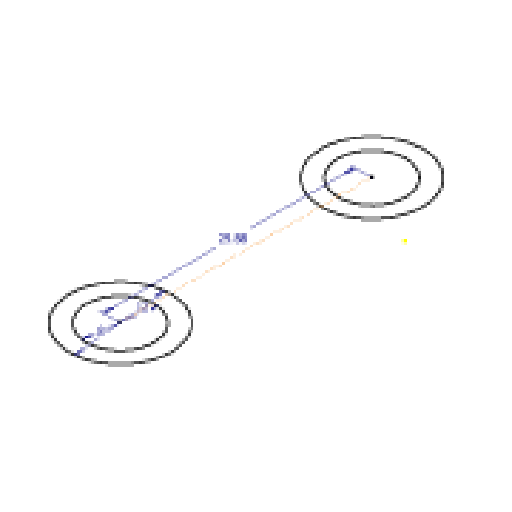
# Autodesk Inventor part: 4barClawSide
Saved by Autodesk Inventor 2023 (Build 270158000, 158)
## iProperties
Created: 2022-10-28
Part Number: 4barClawSide
Material: Generic
Document SubType Name: Modeling
Designer: deli
Density: 1 g/cm^3
Appearance: Default
Author: deli
Autodesk Inventor part; units mm, degrees
ref_plane "YZ Plane" through (0, 0, 0) normal (1, 0, 0) x (0, 1, 0)
ref_plane "XZ Plane" through (0, 0, 0) normal (0, 1, 0) x (-1, 0, 0)
ref_plane "XY Plane" through (0, 0, 0) normal (0, 0, 1) x (1, 0, 0)
sketch "Sketch1" plane through (0, 0, 0) normal (0, 1, 0) x (-1, 0, 0)
  circle A0 centre (8.4569, 15.4658) radius 4
  circle A1 centre (8.4569, -4.5342) radius 4
  arc A2 (14.4569, 15.4658) -> (2.4569, 15.4658) centre (8.4569, 15.4658) ccw
  arc A3 (2.4569, -4.5342) -> (14.4569, -4.5342) centre (8.4569, -4.5342) ccw
  line L0 (8.4569, 15.4658) -> (8.4569, -4.5342) construction
  line L1 (14.4569, 15.4658) -> (14.4569, -4.5342)
  line L2 (2.4569, -4.5342) -> (2.4569, 15.4658)
  point P0 (0, 0)
  dimension "d0" = 8
  dimension "d2" = 12
  dimension "d3" = 20
  constraints: 6 end point, 4 centre point, 4 point on circle, 2 coincident, 2 equal radius, 2 vertical, 1 parallel
  measures "d0" diameter of A0
  measures "d2" diameter of A2
  measures "d3" distance of L0.start L0.end
extrude "Extrusion1" add sketch "Sketch1" along normal blind 20
sketch "Sketch2" plane through (0, 20, 0) normal (0, 1, 0) x (1, 0, 0)
  line L0 (-14.4569, 4.5342) -> (-14.4569, -15.4658) projected
  arc A0 (-14.4569, -15.4658) -> (-2.4569, -15.4658) centre (-8.4569, -15.4658) ccw projected
  line L1 (-2.4569, -15.4658) -> (-2.4569, 4.5342) projected
  arc A1 (-2.4569, 4.5342) -> (-14.4569, 4.5342) centre (-8.4569, 4.5342) ccw projected
  point P0 (0, 0)
extrude "Extrusion2" add sketch "Sketch2" along normal blind 2
sketch "Sketch3" plane through (-2.4569, 0, 15.4658) normal (1, 0, 0) x (0, 0, -1)
  circle A0 centre (10, 12) radius 5
  line L0 (0, 0) -> (0, 22) projected
  line L1 (20, 0) -> (20, 22) projected
  circle A1 centre (10, 12) radius 7 construction
  line L2 (0, 22) -> (20, 22) projected
  point P0 (15.4658, 0)
  dimension "d8" = 10
  dimension "d9" = 10
  dimension "d10" = 20
  dimension "d11" = 14
  dimension "d13" = 10
  constraints: 2 centre point, 1 coincident
  measures "d8" diameter of A0
  measures "d9" distance from line of L0 A0.centre
  measures "d10" distance between parallel lines of L1 L0
  measures "d11" diameter of A1
  measures "d13" distance from line of L2 A0.centre
extrude "Extrusion3" cut sketch "Sketch3" against normal blind 12
sketch "Sketch4" plane through (-2.4569, 0, 15.4658) normal (1, 0, 0) x (0, 0, -1)
  circle A0 centre (10, 12) radius 5 construction
  circle A1 centre (10, 12) radius 6.125
  point P0 (15.4658, 0)
  dimension "d16" = 12.25
  constraints: 1 centre point, 1 coincident
  measures "d16" diameter of A1
extrude "Extrusion4" cut sketch "Sketch4" against normal blind 3.5
sketch "Sketch5" plane through (-14.4569, 0, -4.5342) normal (-1, 0, 0) x (0, 0, 1)
  circle A0 centre (10, 12) radius 6.125 projected
  point P0 (4.5342, 0)
extrude "Extrusion5" cut sketch "Sketch5" against normal blind 3.5
sketch "Sketch6" plane through (-2.4569, 0, 15.4658) normal (1, 0, 0) x (0, 0, -1)
  circle A0 centre (10, 12) radius 6.125 construction
  circle A1 centre (10, 12) radius 7
  point P0 (15.4658, 0)
  dimension "d21" = 14
  constraints: 1 centre point, 1 coincident
  measures "d21" diameter of A1
extrude "Extrusion6" cut sketch "Sketch6" against normal blind 1
sketch "Sketch7" plane through (-14.4569, 0, -4.5342) normal (-1, 0, 0) x (0, 0, 1)
  circle A0 centre (10, 12) radius 7 projected
  point P0 (4.5342, 0)
extrude "Extrusion7" cut sketch "Sketch7" against normal blind 1
equation "\"d9\" = 0.5 * d10"
body "Solid1"
